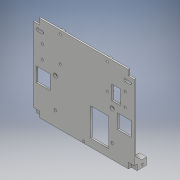
# Autodesk Inventor part: baseplate_jetson_core
Saved by Autodesk Inventor 2018 (Build 220112000, 112)
## iProperties
Created: 2018-05-14
Part Number: baseplate_jetson_core
Material: Generic
Document SubType Name: Modeling
Designer: bitbots
Density: 1 g/cm^3
Appearance: Default
Author: bitbots
Autodesk Inventor part; units mm, degrees
ref_plane "YZ Plane" through (0, 0, 0) normal (1, 0, 0) x (0, 1, 0)
ref_plane "XZ Plane" through (0, 0, 0) normal (0, 1, 0) x (-1, 0, 0)
ref_plane "XY Plane" through (0, 0, 0) normal (0, 0, 1) x (1, 0, 0)
sketch "Sketch1" plane through (0, 0, 0) normal (0, 1, 0) x (-1, 0, 0)
  line L0 (-70, 60) -> (70, 60)
  line L1 (70, 60) -> (70, -60)
  line L2 (70, -60) -> (-70, -60)
  line L3 (-70, -60) -> (-70, 60)
  line L4 (-70, 60) -> (70, -60) construction
  line L5 (70, 60) -> (-70, -60) construction
  point P0 (0, 0)
  dimension "d0" = 140
  dimension "d1" = 120
  constraints: 12 end point, 2 midpoint, 2 parallel, 1 horizontal, 1 perpendicular
  measures "d0" distance of L1.end L2.end
  measures "d1" distance of L0.end L1.end
extrude "Extrusion1" add sketch "Sketch1" along normal blind 2
sketch "Sketch2" plane through (0, 2, 0) normal (0, 1, 0) x (1, 0, 0)
  line L0 (0, 0) -> (0, -2) construction
  line L1 (0, -2) -> (39.5, -2) construction
  line L2 (39.5, -2) -> (-39.5, -2) construction
  line L3 (-39.5, -2) -> (-39.5, 40) construction
  line L4 (-39.5, 40) -> (39.5, 40) construction
  line L5 (39.5, 40) -> (39.5, -2) construction
  circle A0 centre (-39.5, 40) radius 1.75
  circle A1 centre (-39.5, -2) radius 1.75
  circle A2 centre (39.5, -2) radius 1.75
  circle A3 centre (39.5, 40) radius 1.75
  line L6 (70, 60) -> (-70, 60) projected
  dimension "d5" = 39.5
  dimension "d6" = 79
  dimension "d7" = 42
  dimension "d8" = 3.5
  dimension "d9" = 3.5
  dimension "d10" = 3.5
  dimension "d11" = 3.5
  dimension "d36" = 20
  constraints: 12 end point, 4 centre point, 4 coincident, 2 parallel, 2 perpendicular, 1 horizontal, 1 vertical
  measures "d5" distance of L0.end L1.end
  measures "d6" distance of L3.end L4.end
  measures "d7" distance of L2.end L3.end
  measures "d8" diameter of A0
  measures "d9" diameter of A1
  measures "d10" diameter of A2
  measures "d11" diameter of A3
  measures "d36" distance between parallel lines of L6 L4
extrude "Extrusion2" cut sketch "Sketch2" against normal through all
sketch "Sketch3" plane through (0, 2, 0) normal (0, 1, 0) x (1, 0, 0)
  line L0 (0, -12) -> (57.5, -12) construction
  line L1 (57.5, -12) -> (-57.5, -12) construction
  line L2 (-57.5, -12) -> (-57.5, -31) construction
  line L3 (-57.5, -31) -> (57.5, -31) construction
  line L4 (57.5, -31) -> (57.5, -12) construction
  circle A0 centre (-57.5, -12) radius 1.5
  circle A1 centre (57.5, -12) radius 1.5
  circle A2 centre (57.5, -31) radius 1.5
  circle A3 centre (-57.5, -31) radius 1.5
  line L5 (0, -19) -> (33, -19) construction
  line L6 (33, -19) -> (-33, -19) construction
  line L7 (-33, -19) -> (-33, -55) construction
  line L8 (-33, -55) -> (33, -55) construction
  line L9 (33, -55) -> (33, -19) construction
  circle A4 centre (-33, -19) radius 1.5
  circle A5 centre (-33, -55) radius 1.5
  circle A6 centre (33, -55) radius 1.5
  circle A7 centre (33, -19) radius 1.5
  circle A8 centre (39.5, -2) radius 1.75 projected
  circle A9 centre (-39.5, -2) radius 1.75 projected
  line L10 (-70, -60) -> (70, -60) projected
  line L11 (70, -60) -> (70, 60) projected
  line L12 (70, 60) -> (-70, 60) projected
  line L13 (-70, 60) -> (-70, -60) projected
  point P0 (0, 0)
  dimension "d15" = 57.5
  dimension "d16" = 115
  dimension "d17" = 19
  dimension "d18" = 3
  dimension "d19" = 3
  dimension "d20" = 3
  dimension "d21" = 3
  dimension "d23" = 33
  dimension "d24" = 66
  dimension "d25" = 36
  dimension "d26" = 3
  dimension "d27" = 3
  dimension "d28" = 3
  dimension "d29" = 3
  dimension "d33" = 7
  dimension "d35" = 5
  constraints: 20 end point, 8 centre point, 8 coincident, 5 parallel, 3 horizontal, 2 perpendicular
  measures "d15" distance of L0.start L0.end
  measures "d16" distance of L3.end L2.end
  measures "d17" distance of L2.end L1.end
  measures "d18" diameter of A0
  measures "d19" diameter of A1
  measures "d20" diameter of A2
  measures "d21" diameter of A3
  measures "d23" distance of L5.start L5.end
  measures "d24" distance of L8.end L7.end
  measures "d25" distance of L7.end L6.end
  measures "d26" diameter of A4
  measures "d27" diameter of A5
  measures "d28" diameter of A6
  measures "d29" diameter of A7
  measures "d33" distance between parallel lines of L6 L1
  measures "d35" distance between parallel lines of L10 L8
extrude "Extrusion3" cut sketch "Sketch3" against normal through all contours A0 | A1 | A2 | A3 | A4 | A5 | A6 | A7
sketch "Sketch4" plane through (0, 2, 0) normal (0, 1, 0) x (1, 0, 0)
  circle A0 centre (-33, -19) radius 1.5 projected
  circle A1 centre (33, -19) radius 1.5 projected
  circle A2 centre (33, -55) radius 1.5 projected
  circle A3 centre (-33, -55) radius 1.5 projected
  circle A4 centre (-33, -19) radius 4
  circle A5 centre (-33, -55) radius 4
  circle A6 centre (33, -55) radius 4
  circle A7 centre (33, -19) radius 4
  point P0 (0, 0)
  dimension "d39" = 8
  dimension "d40" = 8
  dimension "d41" = 8
  dimension "d42" = 8
  constraints: 4 centre point, 4 coincident
  measures "d39" diameter of A4
  measures "d40" diameter of A5
  measures "d41" diameter of A6
  measures "d42" diameter of A7
extrude "Extrusion4" add sketch "Sketch4" along normal blind 2.6
sketch "Sketch6" plane through (0, 2, 0) normal (0, 1, 0) x (1, 0, 0)
  circle A0 centre (33, -55) radius 4 projected
  circle A1 centre (-33, -19) radius 4 projected
  circle A2 centre (-33, -55) radius 4 projected
  circle A3 centre (33, -19) radius 4 projected
  circle A4 centre (57.5, -31) radius 1.5 projected
  circle A5 centre (-57.5, -12) radius 1.5 projected
  circle A6 centre (57.5, -12) radius 1.5 projected
  circle A7 centre (-57.5, -31) radius 1.5 projected
  circle A8 centre (39.5, -2) radius 1.75 projected
  circle A9 centre (-39.5, 40) radius 1.75 projected
  circle A10 centre (-39.5, -2) radius 1.75 projected
  circle A11 centre (39.5, 40) radius 1.75 projected
  line L0 (-70, -60) -> (70, -60) projected
  line L1 (70, -60) -> (70, 60) projected
  line L2 (70, 60) -> (-70, 60) projected
  line L3 (-70, 60) -> (-70, -60) projected
  line L4 (70, 60) -> (70, -60) projected
  line L5 (70, 60) -> (60, 60)
  line L6 (60, 60) -> (60, 50)
  line L7 (60, 50) -> (70, 50)
  line L8 (70, 50) -> (70, 60)
  point P0 (0, 0)
  dimension "d49" = 10
  dimension "d50" = 10
  constraints: 8 end point, 2 parallel, 1 horizontal, 1 perpendicular
  measures "d49" distance of L7.end L6.end
  measures "d50" distance of L6.end L5.end
extrude "Extrusion6" add sketch "Sketch6" along normal blind 15 contours L7 L6 L2 L1
sketch "Sketch8" plane through (70, 0, 60) normal (1, 0, 0) x (0, 0, -1)
  line L0 (120, 0) -> (0, 0) projected
  line L1 (120, 0) -> (120, 17) projected
  line L2 (110, 17) -> (120, 17) projected
  line L3 (110, 2) -> (110, 17) projected
  line L4 (0, 2) -> (110, 2) projected
  line L5 (0, 0) -> (0, 2) projected
  line L6 (110, 2) -> (110, 11)
  line L7 (110, 2) -> (110, 17) projected
  line L8 (110, 11) -> (116, 11)
  circle A0 centre (116, 11) radius 1.5
  point P0 (60, 0)
  dimension "d56" = 9
  dimension "d57" = 6
  dimension "d58" = 3
  constraints: 4 end point, 1 centre point, 1 coincident, 1 perpendicular, 1 point on line
  measures "d56" distance of L3.start L6.end
  measures "d57" distance of L6.end L8.end
  measures "d58" diameter of A0
extrude "Extrusion8" cut sketch "Sketch8" against normal blind 10 contours A0
mirror "Mirror1" about plane through (0, 0, 0) normal (1, 0, 0) of "Extrusion6", "Extrusion8"
ref_plane "Work Plane1" through (65, 0, 60) normal (1, 0, 0) x (0, 0, -1)
sketch "Sketch11" plane through (65, 0, 60) normal (1, 0, 0) x (0, 0, -1)
  circle A0 centre (116, 11) radius 1.5 projected
  circle A1 centre (116, 11) radius 1.5 projected
  circle A2 centre (116, 11) radius 1.5 projected
  line L0 (116, 11) -> (113.2, 11)
  circle A3 centre (116, 11) radius 1.5 projected
  line L1 (113.2, 12.6166) -> (116, 14.2332)
  line L2 (116, 14.2332) -> (118.8, 12.6166)
  line L3 (118.8, 12.6166) -> (118.8, 9.3834)
  line L4 (118.8, 9.3834) -> (116, 7.7668)
  line L5 (116, 7.7668) -> (113.2, 9.3834)
  line L6 (113.2, 9.3834) -> (113.2, 12.6166)
  line L7 (113.2, 11) -> (118.6, 11)
  line L8 (118.6, 11) -> (118.6, 18.8846)
  line L9 (118.6, 18.8846) -> (113.2, 18.8846)
  line L10 (113.2, 18.8846) -> (113.2, 11)
  point P0 (60, 0)
  dimension "d80" = 2.8
  constraints: 22 end point, 2 horizontal, 2 parallel, 1 coincident, 1 midpoint, 1 perpendicular, 13 other
  measures "d80" distance of L0.start L0.end
extrude "Extrusion11" cut sketch "Sketch11" along normal mid plane 3 contours L7 L8 L2 L3 L4 L5 L6 L0 A0 | A0 L0 L6 L1 L2 L8 L7 | L2 L1 L10 L9 L8
mirror "Mirror2" about plane through (0, 0, 0) normal (1, 0, 0) of "Extrusion11"
chamfer "Chamfer1" distance 8 angle 45 4 edges at (-60, 2, -55) (60, 2, -55) (-65, 2, -50) (65, 2, -50)
sketch "Sketch9" plane through (0, 0, 0) normal (0, -1, 0) x (1, 0, 0)
  circle A0 centre (33, 55) radius 1.5 projected
  circle A1 centre (-33, 19) radius 1.5 projected
  circle A2 centre (57.5, 31) radius 1.5 projected
  circle A3 centre (-57.5, 12) radius 1.5 projected
  circle A4 centre (57.5, 12) radius 1.5 projected
  circle A5 centre (-57.5, 31) radius 1.5 projected
  circle A6 centre (-33, 55) radius 1.5 projected
  circle A7 centre (33, 19) radius 1.5 projected
  circle A8 centre (39.5, 2) radius 1.75 projected
  circle A9 centre (-39.5, -40) radius 1.75 projected
  circle A10 centre (-39.5, 2) radius 1.75 projected
  circle A11 centre (39.5, -40) radius 1.75 projected
  line L0 (70, 60) -> (-70, 60) projected
  line L1 (-70, 60) -> (-70, -60) projected
  line L2 (-70, -60) -> (70, -60) projected
  line L3 (70, -60) -> (70, 60) projected
  line L4 (-70, 60) -> (-70, -60) projected
  line L5 (-70, -60) -> (-62, -60)
  line L6 (-62, -60) -> (-62, -52)
  line L7 (-62, -52) -> (-70, -52)
  line L8 (-70, -52) -> (-70, -60)
  line L9 (70, -60) -> (60, -60) projected
  line L10 (70, -60) -> (60, -60)
  line L11 (70, -50) -> (70, -60)
  line L12 (70, 60) -> (62, 60)
  line L13 (62, 60) -> (62, 52)
  line L14 (62, 52) -> (70, 52)
  line L15 (70, 52) -> (70, 60)
  line L16 (70, 60) -> (-70, 60) projected
  line L17 (-70, 60) -> (-62, 60)
  line L18 (-62, 60) -> (-62, 52)
  line L19 (-62, 52) -> (-70, 52)
  line L20 (-70, 52) -> (-70, 60)
  line L21 (70, -60) -> (62, -60)
  line L22 (62, -60) -> (62, -52)
  line L23 (62, -52) -> (70, -52)
  line L24 (70, -52) -> (70, -60)
  point P0 (0, 0)
  dimension "d64" = 8
  dimension "d65" = 8
  dimension "d68" = 8
  dimension "d69" = 8
  dimension "d70" = 8
  dimension "d71" = 8
  dimension "d96" = 8
  dimension "d97" = 8
  constraints: 36 end point, 8 parallel, 5 horizontal, 4 perpendicular
  measures "d64" distance of L7.end L6.end
  measures "d65" distance of L6.end L5.end
  measures "d68" distance of L14.end L13.end
  measures "d69" distance of L13.end L12.end
  measures "d70" distance of L18.end L19.end
  measures "d71" distance of L17.end L18.end
  measures "d96" distance of L22.end L23.end
  measures "d97" distance of L21.end L22.end
extrude "Extrusion9" cut sketch "Sketch9" against normal blind 4 contours L3 L14 L13 L0 | L18 L19 L1 L0 | L3 L2 L22 L23 | L7 L6 L2 L1
sketch "Sketch10" plane through (0, 2, 0) normal (0, 1, 0) x (1, 0, 0)
  line L0 (-62, -60) -> (62, -60) projected
  line L1 (70, -52) -> (70, 42) projected
  line L2 (52, 42) -> (70, 42) projected
  line L3 (52, 60) -> (52, 42) projected
  line L4 (52, 60) -> (-52, 60) projected
  line L5 (-52, 42) -> (-52, 60) projected
  line L6 (-70, 42) -> (-52, 42) projected
  line L7 (-70, 42) -> (-70, -52) projected
  circle A0 centre (33, -55) radius 4 projected
  circle A1 centre (-33, -19) radius 4 projected
  circle A2 centre (-33, -55) radius 4 projected
  circle A3 centre (33, -19) radius 4 projected
  circle A4 centre (57.5, -31) radius 1.5 projected
  circle A5 centre (-57.5, -12) radius 1.5 projected
  circle A6 centre (57.5, -12) radius 1.5 projected
  circle A7 centre (-57.5, -31) radius 1.5 projected
  circle A8 centre (39.5, -2) radius 1.75 projected
  circle A9 centre (-39.5, 40) radius 1.75 projected
  circle A10 centre (-39.5, -2) radius 1.75 projected
  circle A11 centre (39.5, 40) radius 1.75 projected
  line L8 (-70, 60) -> (70, 60) projected
  line L9 (0, 60) -> (0, 57.5)
  circle A12 centre (0, 57.5) radius 1.5
  line L10 (62, -52) -> (70, -52) projected
  line L11 (-70, -52) -> (-62, -52) projected
  line L12 (-62, -52) -> (-62, -60) projected
  line L13 (62, -60) -> (62, -52) projected
  point P0 (0, 0)
  point P1 (-62, 60)
  point P2 (60, 60)
  dimension "d74" = 2.5
  dimension "d75" = 3
  constraints: 2 end point, 1 centre point, 1 coincident, 1 midpoint, 1 vertical
  measures "d74" distance of L9.start L9.end
  measures "d75" diameter of A12
extrude "Extrusion10" cut sketch "Sketch10" against normal blind 4 contours A12
sketch "Sketch12" plane through (0, 2, 0) normal (0, 1, 0) x (1, 0, 0)
  circle A0 centre (0, 57.5) radius 1.5 projected
  line L0 (-62, -60) -> (62, -60) projected
  line L1 (70, -52) -> (70, 42) projected
  line L2 (52, 42) -> (70, 42) projected
  line L3 (52, 60) -> (52, 42) projected
  line L4 (52, 60) -> (-52, 60) projected
  line L5 (-52, 42) -> (-52, 60) projected
  line L6 (-70, 42) -> (-52, 42) projected
  line L7 (-70, 42) -> (-70, -52) projected
  circle A1 centre (33, -55) radius 4 projected
  circle A2 centre (-33, -19) radius 4 projected
  circle A3 centre (-33, -55) radius 4 projected
  circle A4 centre (33, -19) radius 4 projected
  circle A5 centre (57.5, -31) radius 1.5 projected
  circle A6 centre (-57.5, -12) radius 1.5 projected
  circle A7 centre (57.5, -12) radius 1.5 projected
  circle A8 centre (-57.5, -31) radius 1.5 projected
  circle A9 centre (39.5, -2) radius 1.75 projected
  circle A10 centre (-39.5, 40) radius 1.75 projected
  circle A11 centre (-39.5, -2) radius 1.75 projected
  circle A12 centre (39.5, 40) radius 1.75 projected
  line L8 (70, -52) -> (70, 42) projected
  line L9 (70, -0.25) -> (50, -0.25)
  line L10 (50, -0.25) -> (50, 19.75)
  line L11 (50, 19.75) -> (70, 19.75)
  line L12 (70, 19.75) -> (70, -0.25)
  line L13 (-70, 42) -> (-70, -52) projected
  line L14 (-70, -0.25) -> (-50, -0.25)
  line L15 (-50, -0.25) -> (-50, 19.75)
  line L16 (-50, 19.75) -> (-70, 19.75)
  line L17 (-70, 19.75) -> (-70, -0.25)
  line L18 (62, -52) -> (70, -52) projected
  line L19 (-70, -52) -> (-62, -52) projected
  line L20 (-62, -52) -> (-62, -60) projected
  line L21 (62, -60) -> (62, -52) projected
  point P0 (0, 0)
  dimension "d83" = 20
  dimension "d84" = 20
  dimension "d85" = 20
  dimension "d86" = 20
  constraints: 16 end point, 4 parallel, 3 point on line, 2 horizontal, 2 perpendicular
  measures "d83" distance of L10.end L11.end
  measures "d84" distance of L9.end L10.end
  measures "d85" distance of L16.end L15.end
  measures "d86" distance of L15.end L14.end
extrude "Extrusion12" cut sketch "Sketch12" against normal blind 3 contours L7 L16 L15 L14 | L9 L10 L11 L1
sketch "Sketch13" plane through (0, 2, 0) normal (0, 1, 0) x (1, 0, 0)
  line L0 (-50, -0.25) -> (-70, -0.25) projected
  line L1 (-70, -0.25) -> (-70, -52) projected
  line L2 (-62, -60) -> (62, -60) projected
  line L3 (70, -52) -> (70, -0.25) projected
  line L4 (70, -0.25) -> (50, -0.25) projected
  line L5 (50, -0.25) -> (50, 19.75) projected
  line L6 (50, 19.75) -> (70, 19.75) projected
  line L7 (70, 19.75) -> (70, 42) projected
  line L8 (52, 42) -> (70, 42) projected
  line L9 (52, 60) -> (52, 42) projected
  line L10 (52, 60) -> (-52, 60) projected
  line L11 (-52, 42) -> (-52, 60) projected
  line L12 (-70, 42) -> (-52, 42) projected
  line L13 (-70, 42) -> (-70, 19.75) projected
  line L14 (-70, 19.75) -> (-50, 19.75) projected
  line L15 (-50, 19.75) -> (-50, -0.25) projected
  circle A0 centre (0, 57.5) radius 1.5 projected
  circle A1 centre (33, -55) radius 4 projected
  circle A2 centre (-33, -19) radius 4 projected
  circle A3 centre (-33, -55) radius 4 projected
  circle A4 centre (33, -19) radius 4 projected
  circle A5 centre (57.5, -31) radius 1.5 projected
  circle A6 centre (-57.5, -12) radius 1.5 projected
  circle A7 centre (57.5, -12) radius 1.5 projected
  circle A8 centre (-57.5, -31) radius 1.5 projected
  circle A9 centre (39.5, -2) radius 1.75 projected
  circle A10 centre (-39.5, 40) radius 1.75 projected
  circle A11 centre (-39.5, -2) radius 1.75 projected
  circle A12 centre (39.5, 40) radius 1.75 projected
  line L16 (-70, -60) -> (-61, -60)
  line L17 (-62, -60) -> (62, -60) projected
  line L18 (-61, -60) -> (-61, -45)
  line L19 (-64.5, -45) -> (-57.5, -45) construction
  line L20 (-64.5, -46.75) -> (-57.5, -46.75)
  line L21 (-57.5, -43.25) -> (-64.5, -43.25)
  arc A13 (-64.5, -43.25) -> (-64.5, -46.75) centre (-64.5, -45) ccw
  arc A14 (-57.5, -46.75) -> (-57.5, -43.25) centre (-57.5, -45) ccw
  line L22 (-70, -52) -> (-62, -52) projected
  line L23 (-62, -52) -> (-62, -60) projected
  line L24 (62, -60) -> (62, -52) projected
  line L25 (62, -52) -> (70, -52) projected
  point P0 (0, 0)
  dimension "d90" = 9
  dimension "d91" = 15
  dimension "d92" = 3.5
  dimension "d93" = 3.5
  constraints: 12 end point, 4 point on circle, 4 tangent, 2 centre point, 1 collinear, 1 horizontal, 1 midpoint, 1 parallel, 1 perpendicular
  measures "d90" distance of L16.start L16.end
  measures "d91" distance of L16.end L18.end
  measures "d92" distance of L18.end L19.end
  measures "d93" diameter of A14
extrude "Extrusion13" cut sketch "Sketch13" against normal blind 3 contours A13 L21 A14 L20
mirror "Mirror3" about plane through (0, 0, 0) normal (1, 0, 0) of "Extrusion13"
sketch "Sketch14" plane through (0, 2, 0) normal (0, 1, 0) x (1, 0, 0)
  circle A0 centre (57.5, -31) radius 1.5 projected
  circle A1 centre (57.5, -12) radius 1.5 projected
  circle A2 centre (-57.5, -12) radius 1.5 projected
  circle A3 centre (-57.5, -31) radius 1.5 projected
  circle A4 centre (57.5, -31) radius 4
  circle A5 centre (57.5, -12) radius 1.5 projected
  circle A6 centre (57.5, -12) radius 4
  circle A7 centre (-57.5, -12) radius 1.5 projected
  circle A8 centre (-57.5, -12) radius 4
  circle A9 centre (-57.5, -31) radius 1.5 projected
  circle A10 centre (-57.5, -31) radius 4
  point P0 (0, 0)
  dimension "d98" = 8
  dimension "d99" = 8
  dimension "d100" = 8
  dimension "d101" = 8
  constraints: 4 centre point, 4 coincident
  measures "d98" diameter of A4
  measures "d99" diameter of A6
  measures "d100" diameter of A8
  measures "d101" diameter of A10
extrude "Extrusion14" add sketch "Sketch14" along normal blind 5
sketch "Sketch15" plane through (0, 2, 0) normal (0, 1, 0) x (1, 0, 0)
  circle A0 centre (-57.5, -12) radius 4 projected
  circle A1 centre (57.5, -31) radius 4 projected
  circle A2 centre (57.5, -12) radius 4 projected
  circle A3 centre (-57.5, -31) radius 4 projected
  arc A4 (57.5, -43.25) -> (57.5, -46.75) centre (57.5, -45) ccw projected
  line L0 (57.5, -43.25) -> (64.5, -43.25) projected
  arc A5 (64.5, -46.75) -> (64.5, -43.25) centre (64.5, -45) ccw projected
  line L1 (64.5, -46.75) -> (57.5, -46.75) projected
  arc A6 (-57.5, -46.75) -> (-57.5, -43.25) centre (-57.5, -45) ccw projected
  line L2 (-57.5, -46.75) -> (-64.5, -46.75) projected
  arc A7 (-64.5, -43.25) -> (-64.5, -46.75) centre (-64.5, -45) ccw projected
  line L3 (-64.5, -43.25) -> (-57.5, -43.25) projected
  circle A8 centre (39.5, 40) radius 1.75 projected
  circle A9 centre (-39.5, -2) radius 1.75 projected
  circle A10 centre (-39.5, 40) radius 1.75 projected
  circle A11 centre (39.5, -2) radius 1.75 projected
  circle A12 centre (33, -19) radius 4 projected
  circle A13 centre (-33, -55) radius 4 projected
  circle A14 centre (-33, -19) radius 4 projected
  circle A15 centre (33, -55) radius 4 projected
  line L4 (-70, 19.75) -> (-50, 19.75) projected
  line L5 (-50, 19.75) -> (-50, -0.25) projected
  line L6 (-50, -0.25) -> (-70, -0.25) projected
  line L7 (-70, -0.25) -> (-70, -52) projected
  line L8 (-70, -52) -> (-62, -52) projected
  line L9 (-62, -52) -> (-62, -60) projected
  line L10 (-62, -60) -> (62, -60) projected
  line L11 (62, -60) -> (62, -52) projected
  line L12 (62, -52) -> (70, -52) projected
  line L13 (70, -52) -> (70, -0.25) projected
  line L14 (70, -0.25) -> (50, -0.25) projected
  line L15 (50, -0.25) -> (50, 19.75) projected
  line L16 (50, 19.75) -> (70, 19.75) projected
  line L17 (70, 19.75) -> (70, 42) projected
  line L18 (52, 42) -> (70, 42) projected
  line L19 (52, 60) -> (52, 42) projected
  line L20 (52, 60) -> (-52, 60) projected
  line L21 (-52, 42) -> (-52, 60) projected
  line L22 (-70, 42) -> (-52, 42) projected
  line L23 (-70, 42) -> (-70, 19.75) projected
  circle A16 centre (0, 57.5) radius 1.5 projected
  circle A17 centre (33, -19) radius 1.5 projected
  line L24 (33, -19) -> (45, -19)
  line L25 (45, -19) -> (45, -21)
  line L26 (40, -28.5) -> (50, -28.5)
  line L27 (50, -28.5) -> (50, -13.5)
  line L28 (50, -13.5) -> (40, -13.5)
  line L29 (40, -13.5) -> (40, -28.5)
  line L30 (40, -28.5) -> (50, -13.5) construction
  line L31 (50, -28.5) -> (40, -13.5) construction
  point P0 (0, 0)
  dimension "d104" = 12
  dimension "d105" = 2
  dimension "d106" = 10
  dimension "d107" = 15
  constraints: 16 end point, 2 horizontal, 2 midpoint, 2 parallel, 2 perpendicular
  measures "d104" distance of L24.start L24.end
  measures "d105" distance of L24.end L25.end
  measures "d106" distance of L28.end L27.end
  measures "d107" distance of L27.end L26.end
extrude "Extrusion15" cut sketch "Sketch15" against normal blind 5 contours L29 L28 L27 L26
sketch "Sketch16" plane through (0, 0, 0) normal (0, -1, 0) x (1, 0, 0)
  line L0 (50, 28.5) -> (50, 13.5) projected
  line L1 (50, 13.5) -> (40, 13.5) projected
  line L2 (40, 13.5) -> (40, 28.5) projected
  line L3 (40, 28.5) -> (50, 28.5) projected
  arc A0 (57.5, 46.75) -> (57.5, 43.25) centre (57.5, 45) ccw projected
  line L4 (57.5, 46.75) -> (64.5, 46.75) projected
  arc A1 (64.5, 43.25) -> (64.5, 46.75) centre (64.5, 45) ccw projected
  line L5 (64.5, 43.25) -> (57.5, 43.25) projected
  arc A2 (-57.5, 43.25) -> (-57.5, 46.75) centre (-57.5, 45) ccw projected
  line L6 (-57.5, 43.25) -> (-64.5, 43.25) projected
  arc A3 (-64.5, 46.75) -> (-64.5, 43.25) centre (-64.5, 45) ccw projected
  line L7 (-64.5, 46.75) -> (-57.5, 46.75) projected
  line L8 (-50, -19.75) -> (-70, -19.75) projected
  line L9 (-70, -19.75) -> (-70, -52) projected
  line L10 (-70, -52) -> (-62, -52) projected
  line L11 (-62, -52) -> (-62, -60) projected
  line L12 (-62, -60) -> (62, -60) projected
  line L13 (62, -60) -> (62, -52) projected
  line L14 (62, -52) -> (70, -52) projected
  line L15 (70, -52) -> (70, -19.75) projected
  line L16 (70, -19.75) -> (50, -19.75) projected
  line L17 (50, -19.75) -> (50, 0.25) projected
  line L18 (50, 0.25) -> (70, 0.25) projected
  line L19 (70, 0.25) -> (70, 52) projected
  line L20 (70, 52) -> (62, 52) projected
  line L21 (62, 52) -> (62, 60) projected
  line L22 (62, 60) -> (-62, 60) projected
  line L23 (-62, 60) -> (-62, 52) projected
  line L24 (-62, 52) -> (-70, 52) projected
  line L25 (-70, 52) -> (-70, 0.25) projected
  line L26 (-70, 0.25) -> (-50, 0.25) projected
  line L27 (-50, 0.25) -> (-50, -19.75) projected
  circle A4 centre (0, -57.5) radius 1.5 projected
  circle A5 centre (33, 55) radius 1.5 projected
  circle A6 centre (-33, 19) radius 1.5 projected
  circle A7 centre (57.5, 31) radius 1.5 projected
  circle A8 centre (-57.5, 12) radius 1.5 projected
  circle A9 centre (57.5, 12) radius 1.5 projected
  circle A10 centre (-57.5, 31) radius 1.5 projected
  circle A11 centre (-33, 55) radius 1.5 projected
  circle A12 centre (33, 19) radius 1.5 projected
  circle A13 centre (39.5, 2) radius 1.75 projected
  circle A14 centre (-39.5, -40) radius 1.75 projected
  circle A15 centre (-39.5, 2) radius 1.75 projected
  circle A16 centre (39.5, -40) radius 1.75 projected
  line L28 (50, 0.25) -> (70, 0.25) projected
  line L29 (70, -19.75) -> (66, -19.75)
  line L30 (66, -19.75) -> (66, 0.25)
  line L31 (66, 0.25) -> (70, 0.25)
  line L32 (70, 0.25) -> (70, -19.75)
  line L33 (-50, -19.75) -> (-70, -19.75) projected
  line L34 (-70, -19.75) -> (-66, -19.75)
  line L35 (-66, -19.75) -> (-66, 0.25)
  line L36 (-66, 0.25) -> (-70, 0.25)
  line L37 (-70, 0.25) -> (-70, -19.75)
  point P0 (0, 0)
  dimension "d110" = 4
  dimension "d111" = 4
  constraints: 16 end point, 4 parallel, 2 horizontal, 2 perpendicular, 2 point on line
  measures "d110" distance of L30.end L31.end
  measures "d111" distance of L36.end L35.end
extrude "Extrusion16" add sketch "Sketch16" against normal up to surface (2 mm away) contours L8 L37 L26 L35 | L16 L30 L18 L32
sketch "Sketch17" plane through (0, 2, 0) normal (0, 1, 0) x (1, 0, 0)
  line L0 (70, -52) -> (70, 42) projected
  line L1 (52, 42) -> (70, 42) projected
  line L2 (52, 60) -> (52, 42) projected
  line L3 (52, 60) -> (-52, 60) projected
  line L4 (-52, 42) -> (-52, 60) projected
  line L5 (-70, 42) -> (-52, 42) projected
  line L6 (-70, 42) -> (-70, -52) projected
  line L7 (-70, -52) -> (-62, -52) projected
  line L8 (-62, -52) -> (-62, -60) projected
  line L9 (-62, -60) -> (62, -60) projected
  line L10 (62, -60) -> (62, -52) projected
  line L11 (62, -52) -> (70, -52) projected
  line L12 (66, -0.25) -> (66, 19.75) projected
  line L13 (66, -0.25) -> (50, -0.25) projected
  line L14 (50, -0.25) -> (50, 19.75) projected
  line L15 (50, 19.75) -> (66, 19.75) projected
  line L16 (50, -13.5) -> (50, -28.5) projected
  line L17 (50, -28.5) -> (40, -28.5) projected
  line L18 (40, -28.5) -> (40, -13.5) projected
  line L19 (40, -13.5) -> (50, -13.5) projected
  circle A0 centre (-57.5, -12) radius 4 projected
  circle A1 centre (57.5, -31) radius 4 projected
  circle A2 centre (57.5, -12) radius 4 projected
  circle A3 centre (-57.5, -31) radius 4 projected
  arc A4 (57.5, -43.25) -> (57.5, -46.75) centre (57.5, -45) ccw projected
  line L20 (57.5, -43.25) -> (64.5, -43.25) projected
  arc A5 (64.5, -46.75) -> (64.5, -43.25) centre (64.5, -45) ccw projected
  line L21 (64.5, -46.75) -> (57.5, -46.75) projected
  arc A6 (-57.5, -46.75) -> (-57.5, -43.25) centre (-57.5, -45) ccw projected
  line L22 (-57.5, -46.75) -> (-64.5, -46.75) projected
  arc A7 (-64.5, -43.25) -> (-64.5, -46.75) centre (-64.5, -45) ccw projected
  line L23 (-64.5, -43.25) -> (-57.5, -43.25) projected
  circle A8 centre (39.5, 40) radius 1.75 projected
  circle A9 centre (-39.5, -2) radius 1.75 projected
  circle A10 centre (-39.5, 40) radius 1.75 projected
  circle A11 centre (39.5, -2) radius 1.75 projected
  circle A12 centre (33, -19) radius 4 projected
  circle A13 centre (-33, -55) radius 4 projected
  circle A14 centre (-33, -19) radius 4 projected
  circle A15 centre (33, -55) radius 4 projected
  line L24 (-66, 19.75) -> (-66, -0.25) projected
  line L25 (-66, 19.75) -> (-50, 19.75) projected
  line L26 (-50, 19.75) -> (-50, -0.25) projected
  line L27 (-50, -0.25) -> (-66, -0.25) projected
  circle A16 centre (0, 57.5) radius 1.5 projected
  line L28 (-50, 19.75) -> (-47, 19.75)
  line L29 (-47, 19.75) -> (-47, -0.25)
  line L30 (-47, -0.25) -> (-50, -0.25)
  line L31 (-50, -0.25) -> (-50, 19.75)
  line L32 (50, -0.25) -> (50, 19.75) projected
  line L33 (50, 19.75) -> (47, 19.75)
  line L34 (47, 19.75) -> (47, -0.25)
  line L35 (47, -0.25) -> (50, -0.25)
  line L36 (50, -0.25) -> (50, 19.75)
  point P0 (0, 0)
  dimension "d114" = 3
  dimension "d115" = 3
  constraints: 16 end point, 4 parallel, 2 horizontal, 2 perpendicular, 1 point on line
  measures "d114" distance of L29.end L30.end
  measures "d115" distance of L35.end L34.end
extrude "Extrusion17" cut sketch "Sketch17" against normal blind 5 contours L35 L34 L33 L14 | L28 L29 L30 L26
sketch "Sketch18" plane through (0, 2, 0) normal (0, 1, 0) x (1, 0, 0)
  circle A0 centre (0, 57.5) radius 1.5 projected
  circle A1 centre (33, -55) radius 4 projected
  circle A2 centre (-33, -19) radius 4 projected
  circle A3 centre (-33, -55) radius 4 projected
  circle A4 centre (33, -19) radius 4 projected
  circle A5 centre (39.5, -2) radius 1.75 projected
  circle A6 centre (-39.5, 40) radius 1.75 projected
  circle A7 centre (-39.5, -2) radius 1.75 projected
  circle A8 centre (39.5, 40) radius 1.75 projected
  arc A9 (-57.5, -46.75) -> (-57.5, -43.25) centre (-57.5, -45) ccw projected
  line L0 (-57.5, -46.75) -> (-64.5, -46.75) projected
  arc A10 (-64.5, -43.25) -> (-64.5, -46.75) centre (-64.5, -45) ccw projected
  line L1 (-64.5, -43.25) -> (-57.5, -43.25) projected
  arc A11 (57.5, -43.25) -> (57.5, -46.75) centre (57.5, -45) ccw projected
  line L2 (57.5, -43.25) -> (64.5, -43.25) projected
  arc A12 (64.5, -46.75) -> (64.5, -43.25) centre (64.5, -45) ccw projected
  line L3 (64.5, -46.75) -> (57.5, -46.75) projected
  circle A13 centre (-57.5, -31) radius 4 projected
  circle A14 centre (57.5, -12) radius 4 projected
  circle A15 centre (57.5, -31) radius 4 projected
  circle A16 centre (-57.5, -12) radius 4 projected
  line L4 (50, -13.5) -> (50, -28.5) projected
  line L5 (50, -28.5) -> (40, -28.5) projected
  line L6 (40, -28.5) -> (40, -13.5) projected
  line L7 (40, -13.5) -> (50, -13.5) projected
  line L8 (66, -0.25) -> (47, -0.25) projected
  line L9 (47, -0.25) -> (47, 19.75) projected
  line L10 (47, 19.75) -> (66, 19.75) projected
  line L11 (66, -0.25) -> (66, 19.75) projected
  line L12 (70, -52) -> (70, 42) projected
  line L13 (52, 42) -> (70, 42) projected
  line L14 (52, 60) -> (52, 42) projected
  line L15 (52, 60) -> (-52, 60) projected
  line L16 (-52, 42) -> (-52, 60) projected
  line L17 (-70, 42) -> (-52, 42) projected
  line L18 (-70, 42) -> (-70, -52) projected
  line L19 (-70, -52) -> (-62, -52) projected
  line L20 (-62, -52) -> (-62, -60) projected
  line L21 (-62, -60) -> (62, -60) projected
  line L22 (62, -60) -> (62, -52) projected
  line L23 (62, -52) -> (70, -52) projected
  line L24 (-47, -0.25) -> (-66, -0.25) projected
  line L25 (-66, 19.75) -> (-66, -0.25) projected
  line L26 (-66, 19.75) -> (-47, 19.75) projected
  line L27 (-47, 19.75) -> (-47, -0.25) projected
  circle A17 centre (39.5, 40) radius 1.75 projected
  line L28 (39.5, 40) -> (9.5, 40)
  line L29 (39.5, 40) -> (34.5, 40)
  line L30 (34.5, 40) -> (34.5, 10)
  line L31 (34.5, 40) -> (34.5, 49)
  line L32 (9.5, 40) -> (9.5, 10)
  line L33 (34.5, 49) -> (9.5, 49)
  line L34 (9.5, 49) -> (9.5, 10)
  line L35 (9.5, 10) -> (34.5, 10)
  line L36 (34.5, 10) -> (34.5, 49)
  point P0 (0, 0)
  dimension "d118" = 30
  dimension "d119" = 5
  dimension "d120" = 30
  dimension "d121" = 9
  constraints: 18 end point, 3 vertical, 2 horizontal, 2 parallel, 1 perpendicular, 1 point on line
  measures "d118" distance of L28.start L28.end
  measures "d119" distance of L28.start L29.end
  measures "d120" distance of L29.end L30.end
  measures "d121" distance of L29.end L31.end
extrude "Extrusion18" cut sketch "Sketch18" against normal blind 5 contours L30 L35 L32 L28 | L28 L34 L33 L31
sketch "Sketch21" plane through (0, 2, 0) normal (0, 1, 0) x (1, 0, 0)
  circle A0 centre (39.5, -2) radius 1.75 projected
  circle A1 centre (39.5, 40) radius 1.75 projected
  circle A2 centre (-39.5, 40) radius 1.75 projected
  circle A3 centre (-39.5, -2) radius 1.75 projected
  circle A4 centre (39.5, -2) radius 1.75 projected
  circle A5 centre (39.5, -2) radius 3.5
  circle A6 centre (39.5, 40) radius 3.5
  circle A7 centre (-39.5, -2) radius 3.5
  circle A8 centre (-39.5, 40) radius 1.75 projected
  circle A9 centre (-39.5, 40) radius 3.5
  point P0 (0, 0)
  dimension "d128" = 7
  dimension "d129" = 7
  dimension "d130" = 7
  dimension "d131" = 7
  constraints: 4 centre point, 4 coincident
  measures "d128" diameter of A5
  measures "d129" diameter of A6
  measures "d130" diameter of A7
  measures "d131" diameter of A9
extrude "Extrusion19" add sketch "Sketch21" along normal blind 13
chamfer "Chamfer2" distance 5 angle 45 4 edges at (36, 2, -40) (36, 2, 2) (-43, 2, 2) (-43, 2, -40)
sketch "Sketch22" plane through (0, 0, 0) normal (0, -1, 0) x (1, 0, 0)
  circle A0 centre (39.5, 2) radius 1.75 projected
  circle A1 centre (-39.5, 2) radius 1.75 projected
  circle A2 centre (39.5, 2) radius 2.8
  circle A3 centre (-39.5, 2) radius 2.8
  point P0 (0, 0)
  dimension "d137" = 5.6
  dimension "d138" = 5.6
  constraints: 2 centre point, 2 coincident
  measures "d137" diameter of A2
  measures "d138" diameter of A3
extrude "Extrusion20" cut sketch "Sketch22" against normal blind 3 contours A1 | A2 | A3
sketch "Sketch23" plane through (0, 2, 0) normal (0, 1, 0) x (1, 0, 0)
  line L0 (70, -52) -> (70, 42) projected
  line L1 (52, 42) -> (70, 42) projected
  line L2 (52, 60) -> (52, 42) projected
  line L3 (52, 60) -> (-52, 60) projected
  line L4 (-52, 42) -> (-52, 60) projected
  line L5 (-70, 42) -> (-52, 42) projected
  line L6 (-70, 42) -> (-70, -52) projected
  line L7 (-70, -52) -> (-62, -52) projected
  line L8 (-62, -52) -> (-62, -60) projected
  line L9 (-62, -60) -> (62, -60) projected
  line L10 (62, -60) -> (62, -52) projected
  line L11 (62, -52) -> (70, -52) projected
  line L12 (50, -13.5) -> (50, -28.5) projected
  line L13 (50, -28.5) -> (40, -28.5) projected
  line L14 (40, -28.5) -> (40, -13.5) projected
  line L15 (40, -13.5) -> (50, -13.5) projected
  circle A0 centre (-57.5, -12) radius 4 projected
  circle A1 centre (57.5, -31) radius 4 projected
  circle A2 centre (57.5, -12) radius 4 projected
  circle A3 centre (-57.5, -31) radius 4 projected
  arc A4 (57.5, -43.25) -> (57.5, -46.75) centre (57.5, -45) ccw projected
  line L16 (57.5, -43.25) -> (64.5, -43.25) projected
  arc A5 (64.5, -46.75) -> (64.5, -43.25) centre (64.5, -45) ccw projected
  line L17 (64.5, -46.75) -> (57.5, -46.75) projected
  arc A6 (-57.5, -46.75) -> (-57.5, -43.25) centre (-57.5, -45) ccw projected
  line L18 (-57.5, -46.75) -> (-64.5, -46.75) projected
  arc A7 (-64.5, -43.25) -> (-64.5, -46.75) centre (-64.5, -45) ccw projected
  line L19 (-64.5, -43.25) -> (-57.5, -43.25) projected
  circle A8 centre (33, -19) radius 4 projected
  circle A9 centre (-33, -55) radius 4 projected
  circle A10 centre (-33, -19) radius 4 projected
  circle A11 centre (33, -55) radius 4 projected
  circle A12 centre (0, 57.5) radius 1.5 projected
  arc A13 (34.5, 33.1261) -> (34.5, 46.8739) centre (39.5, 40) ccw projected
  line L20 (34.5, 33.1261) -> (34.5, 10) projected
  line L21 (34.5, 10) -> (9.5, 10) projected
  line L22 (9.5, 10) -> (9.5, 49) projected
  line L23 (9.5, 49) -> (34.5, 49) projected
  line L24 (34.5, 49) -> (34.5, 46.8739) projected
  arc A14 (47, 2) -> (47.8179, -0.25) centre (39.5, -2) ccw projected
  line L25 (47, 2) -> (47, 19.75) projected
  line L26 (47, 19.75) -> (66, 19.75) projected
  line L27 (66, -0.25) -> (66, 19.75) projected
  line L28 (66, -0.25) -> (47.8179, -0.25) projected
  arc A15 (-47.8179, -0.25) -> (-47, 2) centre (-39.5, -2) ccw projected
  line L29 (-47.8179, -0.25) -> (-66, -0.25) projected
  line L30 (-66, 19.75) -> (-66, -0.25) projected
  line L31 (-66, 19.75) -> (-47, 19.75) projected
  line L32 (-47, 19.75) -> (-47, 2) projected
  circle A16 centre (-39.5, 40) radius 8.5 projected
  line L33 (39, -31) -> (51, -31)
  line L34 (51, -31) -> (51, -11)
  line L35 (51, -11) -> (39, -11)
  line L36 (39, -11) -> (39, -31)
  line L37 (39, -31) -> (51, -11) construction
  line L38 (51, -31) -> (39, -11) construction
  point P0 (0, 0)
  point P1 (45, -21)
  dimension "d141" = 12
  dimension "d142" = 20
  constraints: 12 end point, 2 midpoint, 2 parallel, 1 horizontal, 1 perpendicular
  measures "d141" distance of L35.end L34.end
  measures "d142" distance of L34.end L33.end
extrude "Extrusion21" cut sketch "Sketch23" against normal blind 10 contours L36 L35 L34 L33
body "Solid1"
